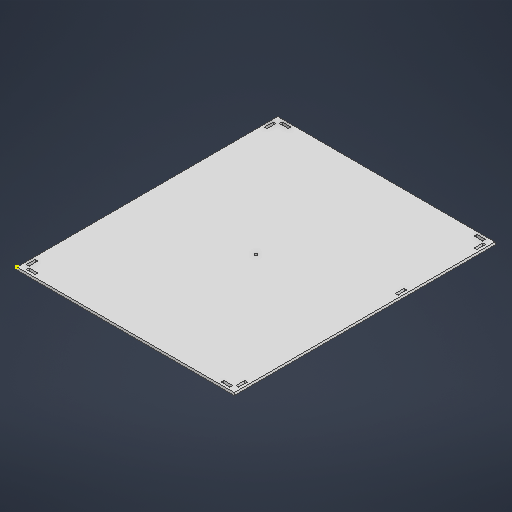
# Autodesk Inventor part: Base_de_equipo
Saved by Autodesk Inventor 2026 (Build 300175000, 175)
## iProperties
Created: 2026-05-15
Part Number: Base_de_equipo
Material: Generic
Document SubType Name: Modeling
Designer: juana
Density: 1 g/cm^3
Appearance: Default
Author: juana
Autodesk Inventor part; units mm, degrees
ref_plane "YZ Plane" through (0, 0, 0) normal (1, 0, 0) x (0, 1, 0)
ref_plane "XZ Plane" through (0, 0, 0) normal (0, 1, 0) x (-1, 0, 0)
ref_plane "XY Plane" through (0, 0, 0) normal (0, 0, 1) x (1, 0, 0)
sketch "Sketch1" plane through (0, 0, 0) normal (0, 1, 0) x (-1, 0, 0)
  line L0 (0, -300) -> (-250, -300)
  line L1 (-250, -300) -> (-250, 0)
  line L2 (-250, 0) -> (0, 0)
  line L3 (0, 0) -> (0, -300)
  dimension "d0" = 300
  dimension "d1" = 250
  constraints: 8 end point, 2 parallel, 1 coincident, 1 horizontal, 1 horizontal alignment, 1 perpendicular
  measures "d0" distance of L2.end L0.start
  measures "d1" distance of L0.start L0.end
extrude "Extrusion1" add sketch "Sketch1" along normal blind 3
sketch "Sketch2" plane through (0, 3, 0) normal (0, 1, 0) x (1, 0, 0)
  line L0 (8, 3) -> (18, 3)
  line L1 (18, 3) -> (18, 6)
  line L2 (18, 6) -> (8, 6)
  line L3 (8, 6) -> (8, 3)
  line L4 (3, 8) -> (3, 18)
  line L5 (3, 18) -> (6, 18)
  line L6 (0, 0) -> (250, 0) construction
  line L7 (0, 300) -> (0, 0) construction
  line L8 (125, 0) -> (125, 300) construction
  line L9 (250, 300) -> (0, 300) construction
  line L10 (0, 150) -> (250, 150) construction
  line L11 (250, 0) -> (250, 300) construction
  line L12 (3, 8) -> (6, 8)
  line L13 (6, 8) -> (6, 18)
  line L14 (242, 3) -> (232, 3)
  line L15 (232, 3) -> (232, 6)
  line L16 (232, 6) -> (242, 6)
  line L17 (242, 6) -> (242, 3)
  line L18 (247, 8) -> (247, 18)
  line L19 (247, 18) -> (244, 18)
  line L20 (247, 8) -> (244, 8)
  line L21 (244, 8) -> (244, 18)
  line L22 (8, 297) -> (18, 297)
  line L23 (18, 297) -> (18, 294)
  line L24 (18, 294) -> (8, 294)
  line L25 (8, 294) -> (8, 297)
  line L26 (3, 292) -> (3, 282)
  line L27 (3, 282) -> (6, 282)
  line L28 (3, 292) -> (6, 292)
  line L29 (6, 292) -> (6, 282)
  line L30 (242, 297) -> (232, 297)
  line L31 (232, 297) -> (232, 294)
  line L32 (242, 294) -> (242, 297)
  line L33 (247, 292) -> (247, 282)
  line L34 (247, 282) -> (244, 282)
  line L35 (247, 292) -> (244, 292)
  line L36 (244, 292) -> (244, 282)
  line L37 (232, 294) -> (242, 294)
  dimension "d6" = 8
  dimension "d7" = 3
  dimension "d9" = 10
  dimension "d12" = 3
  dimension "d13" = 10
  dimension "d14" = 3
  dimension "d15" = 3
  dimension "d16" = 8
  constraints: 68 end point, 24 symmetric about line, 4 midpoint, 3 horizontal, 2 parallel, 2 vertical, 1 perpendicular
  measures "d6" distance from line of L6.start L3
  measures "d7" distance from line of L6.start L0
  measures "d9" distance of L4.start L4.end
  measures "d12" distance of L2.end L0.start
  measures "d13" distance of L0.start L0.end
  measures "d14" distance of L4.start L12.end
  measures "d15" distance between parallel lines of L7 L4
  measures "d16" distance between parallel lines of L6 L12
extrude "Extrusion2" cut sketch "Sketch2" against normal blind 10
sketch "Sketch3" plane through (0, 3, 0) normal (0, 1, 0) x (1, 0, 0)
  circle A0 centre (125, 150) radius 1.5
  line L0 (0, 300) -> (0, 0) projected
  line L1 (0, 0) -> (250, 0) projected
  point P0 (0, 150)
  point P1 (125, 0)
  dimension "d17" = 3
  constraints: 2 midpoint, 1 centre point, 1 horizontal alignment, 1 vertical alignment
  measures "d17" diameter of A0
extrude "Extrusion3" cut sketch "Sketch3" against normal blind 3
sketch "Sketch4" plane through (0, 3, 0) normal (0, 1, 0) x (1, 0, 0)
  line L0 (141.42, 3) -> (151.42, 3)
  line L1 (151.42, 3) -> (151.42, 6)
  line L2 (151.42, 6) -> (141.42, 6)
  line L3 (141.42, 6) -> (141.42, 3)
  line L4 (232, 3) -> (232, 6) projected
  line L5 (247, 201.42) -> (244, 201.42)
  line L6 (244, 201.42) -> (244, 191.42)
  line L7 (244, 191.42) -> (247, 191.42)
  line L8 (247, 191.42) -> (247, 201.42)
  point P0 (0, 0)
  point P1 (247, 282)
  dimension "d20" = 3
  dimension "d21" = 80.58
  dimension "d22" = 10
  dimension "d25" = 10
  dimension "d26" = 80.58
  dimension "d27" = 3
  constraints: 16 end point, 4 parallel, 2 horizontal, 2 perpendicular, 1 horizontal alignment, 1 vertical alignment
  measures "d20" distance of L2.end L0.start
  measures "d21" distance between parallel lines of L4 L1
  measures "d22" distance of L1.end L2.end
  measures "d25" distance of L5.end L6.end
  measures "d26" distance from line of point (247, 282) L5
  measures "d27" distance of L6.end L7.end
extrude "Extrusion4" cut sketch "Sketch4" against normal blind 3 contours L8 L7 L6 L5
sketch "Sketch5" plane through (0, 3, 0) normal (0, 1, 0) x (1, 0, 0)
  point P0 (0, 0)
equation "\"d10\" = d4"
equation "\"d4\" = 10"
body "Solid1"
